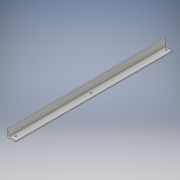
# Autodesk Inventor part: Part2
Saved by Autodesk Inventor 2017 (Build 210142000, 142)
## iProperties
Created: 2018-10-17
Part Number: Part2
Material: Generic
Document SubType Name: Modeling
Designer: ddeboer
Density: 1 g/cm^3
Appearance: Default
Author: ddeboer
Autodesk Inventor part; units mm, degrees
ref_plane "YZ Plane" through (0, 0, 0) normal (1, 0, 0) x (0, 1, 0)
ref_plane "XZ Plane" through (0, 0, 0) normal (0, 1, 0) x (-1, 0, 0)
ref_plane "XY Plane" through (0, 0, 0) normal (0, 0, 1) x (1, 0, 0)
sketch "Sketch1" plane through (0, 0, 0) normal (0, 0, 1) x (1, 0, 0)
  line L0 (0, 25.4) -> (0, 1.778)
  line L1 (1.778, 0) -> (25.4, 0)
  line L2 (3.175, 25.4) -> (3.175, 4.953)
  line L3 (4.953, 3.175) -> (25.4, 3.175)
  line L4 (0, 25.4) -> (3.175, 25.4)
  line L5 (25.4, 3.175) -> (25.4, 0)
  arc A0 (3.175, 4.953) -> (4.953, 3.175) centre (4.953, 4.953) ccw
  arc A1 (0, 1.778) -> (1.778, 0) centre (1.778, 1.778) ccw
  point P0 (0, 0)
  point P1 (3.175, 3.175)
  dimension "d0" = 25.4
  dimension "d1" = 25.4
  dimension "d2" = 3.175
  dimension "d21" = 1.778
  constraints: 12 end point, 4 point on circle, 4 point on line, 4 tangent, 2 centre point, 2 perpendicular, 2 vertical, 1 equal radius, 1 horizontal, 1 other
  measures "d0" distance of L0.start point (0, 0)
  measures "d1" distance of point (0, 0) L1.end
  measures "d2" distance between parallel lines of L2 L0
  measures "d21" radius of A0
extrude "Extrusion1" add sketch "Sketch1" along normal blind 495.3
sketch "Sketch2" plane through (3.175, 3.175, 0) normal (0, 1, 0) x (1, 0, 0)
  circle A0 centre (9.525, -482.6) radius 2.8398
  line L0 (22.225, -495.3) -> (1.778, -495.3) projected
  line L1 (22.225, 0) -> (22.225, -495.3) projected
  circle A1 centre (9.525, -6.35) radius 2.8398
  point P0 (-3.175, 0)
  point P1 (0, -501.65)
  point P2 (1.778, -495.3)
  dimension "d5" = 12.7
  dimension "d6" = 12.7
  dimension "d9" = 476.25
  constraints: 2 centre point, 1 vertical, 3 other
  measures "d6" distance from line of A0.centre L1
  measures "d9" distance of A0.centre A1.centre
hole "Hole1" at (12.7, 3.175, 482.6) at (12.7, 3.175, 6.35) direction (0, -1, 0) diameter 5.1054 depth 25.4 tip angle 118 clearance for "Flat Head Machine Screw (82)" size "#10" standard "Ansi Unified Screw Threads"
sketch "Sketch5" plane through (4.953, 3.175, 0) normal (0, 1, 0) x (1, 0, 0)
  circle A0 centre (7.747, -482.6) radius 2.5527 projected
  circle A1 centre (7.747, -6.35) radius 2.5527 projected
  line L0 (7.747, -482.6) -> (7.747, -6.35) construction
  circle A2 centre (7.747, -244.475) radius 2.5527
  point P0 (-4.953, 0)
  constraints: 2 end point, 1 centre point, 1 midpoint, 1 vertical
hole "Hole2" at (12.7, 3.175, 244.475) direction (0, -1, 0) diameter 5.1054 depth 25.4 tip angle 118 clearance for "Flat Head Machine Screw (82)" size "#10" standard "Ansi Unified Screw Threads"
body "Solid1"
